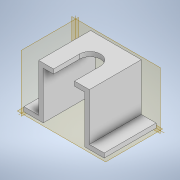
# Autodesk Inventor part: Bridge
Saved by Autodesk Inventor 2022 (Build 260153000, 153)
## iProperties
Created: 2022-05-11
Part Number: Bridge
Material: Generic
Document SubType Name: Modeling
Designer: dovalle
Density: 1 g/cm^3
Appearance: Default
Author: dovalle
Autodesk Inventor part; units mm, degrees
sketch "Sketch1" plane through (0, 0, 0) normal (0, 0, 1) x (1, 0, 0)
  line L0 (0, 0) -> (0, 3)
  line L1 (0, 3) -> (10, 3)
  line L2 (10, 3) -> (10, 35)
  line L3 (10, 35) -> (44.15, 35)
  line L4 (44.15, 35) -> (44.15, 3)
  line L5 (44.15, 3) -> (54.15, 3)
  line L6 (54.15, 3) -> (54.15, 0)
  line L7 (54.15, 0) -> (41.15, 0)
  line L8 (41.15, 0) -> (41.15, 32)
  line L9 (41.15, 32) -> (13, 32)
  line L10 (13, 32) -> (13, 0)
  line L11 (13, 0) -> (0, 0)
  constraints: 24 end point, 7 perpendicular, 3 point on line, 1 parallel, 1 vertical
extrude "Extrusion1" add sketch "Sketch1" along normal blind 35
sketch "Sketch2" plane through (10, 35, 0) normal (0, 1, 0) x (1, 0, 0)
  arc A0 (24.15, -17.5) -> (10, -17.5) centre (17.075, -17.5) ccw
  line L0 (10, -17.5) -> (10, -35)
  line L1 (34.15, -17.5) -> (34.15, -35)
  line L2 (24.15, -17.5) -> (24.15, -35)
  line L3 (10, -35) -> (24.15, -35)
  line L4 (3, -35) -> (31.15, -35) projected
  point P0 (0, 0)
  point P1 (34.15, 0)
  point P2 (0, -35)
  constraints: 8 end point, 2 point on circle, 1 centre point, 1 collinear, 1 tangent, 1 vertical
extrude "Extrusion2" cut sketch "Sketch2" against normal blind 10
body "Solid1"
